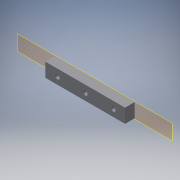
# Autodesk Inventor part: bumper lever support
Saved by Autodesk Inventor 2016 (Build 200138000, 138)
## iProperties
Created: 2015-09-30
Part Number: bumper lever support
Material: Generic
Document SubType Name: Modeling
Designer: Jesse Stevenson
Density: 1 g/cm^3
Appearance: Default
Author: Jesse Stevenson
Autodesk Inventor part; units mm, degrees
ref_plane "YZ Plane" through (0, 0, 0) normal (1, 0, 0) x (0, 1, 0)
ref_plane "XZ Plane" through (0, 0, 0) normal (0, 1, 0) x (-1, 0, 0)
ref_plane "XY Plane" through (0, 0, 0) normal (0, 0, 1) x (1, 0, 0)
ref_plane "Work Plane1" through (0, 0, 0.5676) normal (0, 0, 1) x (1, 0, 0)
sketch "Sketch1" plane through (0, 0, 0.5676) normal (0, 0, 1) x (1, 0, 0)
  circle A0 centre (19.2786, 3.175) radius 1.0541 projected
  circle A1 centre (44.6786, 3.175) radius 1.0541 projected
  circle A2 centre (57.3786, 3.175) radius 1.0541 construction
  circle A3 centre (6.5786, 3.175) radius 1.0541 construction
  circle A4 centre (31.9786, 3.175) radius 1.0541 projected
  line L0 (0, 0) -> (63.9572, 0) construction
  line L1 (63.9572, 0) -> (63.9572, 6.35) construction
  line L2 (0, 6.35) -> (63.9572, 6.35) construction
  line L3 (0, 0) -> (0, 6.35) construction
  line L4 (46.3859, 6.35) -> (17.5713, 6.35)
  line L5 (17.5713, 6.35) -> (17.5713, 0)
  line L6 (17.5713, 0) -> (46.3859, 0)
  line L7 (46.3859, 0) -> (46.3859, 6.35)
  line L8 (44.6786, 3.175) -> (46.3859, 3.175) construction
  line L9 (19.2786, 3.175) -> (17.5713, 3.175) construction
  constraints: 12 end point, 2 midpoint, 2 parallel, 2 point on line, 1 collinear, 1 horizontal, 1 perpendicular
extrude "Extrusion1" add sketch "Sketch1" along normal blind 4.318
sketch "Sketch2" plane through (17.5713, 0, 0.5676) normal (0, -1, 0) x (1, 0, 0)
  line L0 (0, 0) -> (28.8145, 0) projected
  line L1 (28.8145, 0) -> (28.8145, 4.318) projected
  line L2 (0, 4.318) -> (28.8145, 4.318) projected
  line L3 (0, 0) -> (0, 4.318) projected
  point P0 (-17.5713, -0.5676)
extrude "Extrusion2" add sketch "Sketch2" along normal blind 4.318
sketch "Sketch3" plane through (0, 0, 4.8856) normal (0, 0, 1) x (1, 0, 0)
  line L0 (46.3859, 6.35) -> (46.3859, -4.318) projected
  line L1 (46.3859, 1.016) -> (17.5713, 1.016)
  line L2 (17.5713, 6.35) -> (17.5713, -4.318) projected
  line L3 (46.3859, -4.318) -> (17.5713, -4.318) projected
  line L4 (46.3859, 1.016) -> (17.5713, 1.016)
  line L5 (17.5713, 1.016) -> (17.5713, -4.318)
  line L6 (17.5713, -4.318) -> (46.3859, -4.318)
  line L7 (46.3859, -4.318) -> (46.3859, 1.016)
  point P0 (0, 0)
  constraints: 10 end point, 2 midpoint, 2 parallel, 1 horizontal, 1 perpendicular
extrude "Extrusion3" add sketch "Sketch3" along normal blind 21.7805
sketch "Sketch4" plane through (17.5713, -4.318, 0.5676) normal (0, -1, 0) x (1, 0, 0)
  line L0 (0, 0) -> (28.8145, 0) construction
  line L1 (28.8145, 0) -> (28.8145, 26.0985) construction
  line L2 (0, 26.0985) -> (28.8145, 26.0985) construction
  line L3 (0, 0) -> (0, 26.0985) construction
  line L4 (0, 26.0985) -> (28.8145, 26.0985) construction
  line L5 (23.0767, 26.0985) -> (17.1743, 18.3371)
  line L6 (12.2917, 18.1299) -> (5.0882, 26.0985)
  line L7 (20.1255, 22.2178) -> (14.4073, 22.2178) construction
  line L8 (14.4073, 22.2178) -> (14.4073, 26.0985) construction
  line L9 (14.4073, 22.2178) -> (8.69, 22.1142) construction
  line L10 (5.0882, 26.0985) -> (23.0767, 26.0985)
  arc A0 (12.2917, 18.1299) -> (17.1743, 18.3371) centre (14.647, 20.259) ccw
  point P0 (-17.5713, -0.5676)
  point P1 (14.8579, 15.2912)
  dimension "d8" = 3.175
  constraints: 12 end point, 4 point on line, 3 midpoint, 2 point on circle, 2 tangent, 1 centre point, 1 collinear, 1 equal length, 1 horizontal, 1 vertical
  measures "d8" radius of A0
extrude "Extrusion4" cut sketch "Sketch4" against normal through all
sketch "Sketch5" plane through (17.5713, -4.318, 0.5676) normal (0, -1, 0) x (1, 0, 0)
  line L0 (23.0767, 26.0985) -> (17.1743, 18.3371) projected
  arc A0 (12.2917, 18.1299) -> (17.1743, 18.3371) centre (14.647, 20.259) ccw projected
  line L1 (12.2917, 18.1299) -> (5.0882, 26.0985) projected
  line L2 (0, 26.0985) -> (5.0882, 26.0985) projected
  line L3 (0, 0) -> (0, 26.0985) projected
  line L4 (0, 0) -> (28.8145, 0) projected
  line L5 (28.8145, 0) -> (28.8145, 26.0985) projected
  line L6 (23.0767, 26.0985) -> (28.8145, 26.0985) projected
  line L7 (28.8145, 0) -> (28.8145, 26.0985) construction
  line L8 (0, 4.318) -> (0, 26.0985) construction
  line L9 (28.8145, 19.7485) -> (0, 19.7485) construction
  line L10 (2.8689, 24.0238) -> (2.8689, 16.2202) construction
  line L11 (23.0767, 26.0985) -> (28.8145, 26.0985) construction
  line L12 (25.9456, 26.0985) -> (25.9456, 15.2083) construction
  line L13 (25.9456, 22.1235) -> (28.8145, 22.1235) construction
  line L14 (28.8145, 4.318) -> (28.8145, 26.0985) construction
  line L15 (2.8689, 22.1235) -> (0, 22.1235) construction
  line L16 (0, 0) -> (0, 26.0985) construction
  circle A1 centre (25.9456, 19.7485) radius 1.7859
  circle A2 centre (2.8689, 19.7485) radius 1.7859
  point P0 (-17.5713, -0.5676)
  dimension "d10" = 6.35
  dimension "d16" = 3.5719
  constraints: 11 point on line, 10 end point, 3 perpendicular, 2 centre point, 2 vertical, 1 collinear, 1 equal radius, 1 midpoint
  measures "d10" distance between parallel lines of L2 L9
  measures "d16" diameter of A1
extrude "Extrusion5" cut sketch "Sketch5" against normal through all contours A1 | A2
sketch "Sketch6" plane through (0, 0, 26.6661) normal (0, 0, 1) x (1, 0, 0)
  line L0 (17.5713, 1.016) -> (17.5713, -4.318) construction
  line L1 (46.3859, -4.318) -> (46.3859, 1.016) construction
  circle A0 centre (31.9786, 3.175) radius 1.0541 construction
  circle A1 centre (44.6786, 3.175) radius 1.0541 construction
  circle A2 centre (19.2786, 3.175) radius 1.0541 construction
  line L2 (46.3859, 6.35) -> (17.5713, 6.35) construction
  line L3 (46.3859, 6.35) -> (46.3859, -4.318) construction
  line L4 (17.5713, -4.318) -> (46.3859, -4.318) construction
  line L5 (17.5713, 6.35) -> (17.5713, -4.318) construction
  line L6 (46.3859, -1.651) -> (17.5713, -1.651)
  line L7 (46.3859, -1.651) -> (17.5713, -1.651)
  line L8 (17.5713, -1.651) -> (17.5713, 6.35)
  line L9 (17.5713, 6.35) -> (46.3859, 6.35)
  line L10 (46.3859, 6.35) -> (46.3859, -1.651)
  point P0 (0, 0)
  constraints: 10 end point, 2 parallel, 2 perpendicular, 2 point on line, 1 horizontal
extrude "Extrusion6" cut sketch "Sketch6" against normal blind 15.4305
fillet "Fillet1" radius 4.7625 3 edges at (17.5713, -2.9845, 26.6661) (17.5713, -1.651, 18.9509) (46.3858, -2.9845, 26.6661)
body "Solid1"
